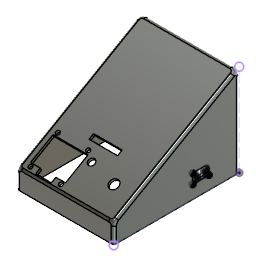
Morse Keyer Top Shell (Autodesk Fusion 360 design; units mm, degrees)
part number: 2026-05-24-21-26-59-922
Autodesk Fusion 360 part; units mm, degrees
sketch "Sketch1" plane through (0, 0, 0) normal (0, 0, 1) x (1, 0, 0)
  line L0 (37.5, 48.5) -> (-37.5, 48.5)
  line L1 (-37.5, 48.5) -> (-37.5, -48.5)
  line L2 (-37.5, -48.5) -> (37.5, -48.5)
  line L3 (37.5, -48.5) -> (37.5, 48.5)
  line L4 (37.5, 48.5) -> (-37.5, -48.5) construction
  line L5 (-37.5, 48.5) -> (37.5, -48.5) construction
  dimension "d1" = 75
  dimension "d2" = 97
  constraint horizontal L0
  constraint perpendicular L0 L1
  constraint parallel L0 L2
  constraint parallel L1 L3
  constraint coincident L4 origin
  constraint coincident L5 origin
  measures "d1" distance of L1.end L2.end
  measures "d2" distance of L0.end L1.end
extrude "Extrude1" add sketch "Sketch1" along normal blind 15
sketch "Sketch2" plane through (37.5, 0, 0) normal (1, 0, 0) x (0, 1, 0)
  line L0 (-48.5, 0) -> (48.5, 0)
  line L1 (48.5, 0) -> (48.5, 15)
  line L2 (48.5, 15) -> (-48.5, 15)
  line L3 (-48.5, 15) -> (-48.5, 0)
  line L4 (-48.5, 15) -> (48.5, 71.003)
  line L5 (-48.5, 15) -> (74.9401, 15) construction
  line L6 (48.5, 71.003) -> (48.5, 15)
  dimension "d5" = 30
  constraint horizontal L5
  constraint coincident L2.end L3.start
  constraint coincident L1.end L2.start
  constraint parallel L1 L6
  measures "d5" angle of L4 L5
extrude "Extrude2" add sketch "Sketch2" against normal up to surface (75 mm away) contours L2 L4 L6
sketch "Sketch3" plane through (0, -18.6202, 32.2511) normal (0, -0.5, 0.866025) x (1, 0, 0)
  line L0 (-37.5, 77.5037) -> (-37.5, -34.5022)
  line L1 (-37.5, -34.5022) -> (37.5, -34.5022)
  line L2 (37.5, -34.5022) -> (37.5, 77.5037)
  line L3 (37.5, 77.5037) -> (-37.5, 77.5037)
  line L4 (11, 3.5037) -> (-11, 3.5037)
  line L5 (-11, 3.5037) -> (-11, -0.4963)
  line L6 (-11, -0.4963) -> (11, -0.4963)
  line L7 (11, -0.4963) -> (11, 3.5037)
  line L8 (11, 3.5037) -> (-11, -0.4963) construction
  line L9 (-11, 3.5037) -> (11, -0.4963) construction
  line L10 (-32, -32.5022) -> (-5, -32.5022)
  line L11 (-5, -32.5022) -> (-5, -8.5022)
  line L12 (-5, -8.5022) -> (-32, -8.5022)
  line L13 (-32, -8.5022) -> (-32, -32.5022)
  circle A0 centre (-30.25, -6.2022) radius 1.5
  circle A1 centre (-6.75, -6.2022) radius 1.5
  circle A2 centre (21.25, -15.4993) radius 3.5
  line L14 (-32, -32.5022) -> (-24.5, -32.5022)
  line L15 (-24.5, -32.5022) -> (-24.5, -28.5022)
  line L16 (-24.5, -28.5022) -> (-32, -28.5022)
  line L17 (-32, -28.5022) -> (-32, -32.5022)
  line L18 (-5, -32.5022) -> (-12.5, -32.5022)
  line L19 (-12.5, -32.5022) -> (-12.5, -28.5022)
  line L20 (-12.5, -28.5022) -> (-5, -28.5022)
  line L21 (-5, -28.5022) -> (-5, -32.5022)
  circle A3 centre (-6.75, -30.5022) radius 1.5
  circle A4 centre (-30.25, -30.5022) radius 1.5
  line L22 (11, 3.5037) -> (37.5, 3.5037) construction
  line L23 (-11, 3.5037) -> (-37.5, 3.5037) construction
  line L24 (21.25, 3.5037) -> (21.25, -34.5022) construction
  circle A5 centre (0, -11.0022) radius 2.5
  line L25 (-5, -8.5022) -> (6, -8.5022) construction
  point P0 (0, 1.5037)
  dimension "d8" = 22
  dimension "d9" = 4
  dimension "d10" = 74
  dimension "d11" = 27
  dimension "d12" = 24
  dimension "d14" = 2
  dimension "d17" = 3
  dimension "d18" = 2.3
  dimension "d20" = 2.3
  dimension "d22" = 7
  dimension "d37" = 3
  dimension "d38" = 7.5
  dimension "d39" = 4
  dimension "d40" = 7.5
  dimension "d41" = 4
  dimension "d42" = 3
  dimension "d43" = 2
  dimension "d44" = 1.75
  dimension "d45" = 23.5
  dimension "d46" = 24.3
  dimension "d54" = 1.75
  dimension "d55" = 1.75
  dimension "d56" = 16.25
  dimension "d57" = 5
  dimension "d58" = 5
  constraint horizontal L4
  constraint perpendicular L4 L5
  constraint parallel L4 L6
  constraint parallel L5 L7
  constraint coincident L8 P0
  constraint coincident L9 P0
  constraint horizontal L10
  constraint vertical L11
  constraint horizontal L12
  constraint vertical L13
  constraint horizontal L14
  constraint vertical L15
  constraint horizontal L16
  constraint vertical L17
  constraint horizontal L18
  constraint vertical L19
  constraint horizontal L20
  constraint vertical L21
  constraint coincident L2 L22.end
  constraint perpendicular L2 L22
  constraint coincident L0 L23.end
  constraint perpendicular L0 L23
  constraint coincident L22 L24.start
  constraint coincident L1 L24.end
  constraint perpendicular L1 L24
  constraint midpoint A2.centre L24
  constraint perpendicular L11 L25
  constraint tangent A5 L25
  measures "d8" distance of L5.end L6.end
  measures "d9" distance of L4.end L5.end
  measures "d10" distance of L3 L4
  measures "d11" distance of L10.start L10.end
  measures "d12" distance of L10.start L12.end
  measures "d14" distance of L1 L10
  measures "d17" diameter of A0
  measures "d18" distance of L12 A0.centre
  measures "d20" distance of L12 A1.centre
  measures "d22" diameter of A2
  measures "d37" diameter of A1
  measures "d38" distance of L10.start L14.end
  measures "d39" distance of L10.start L16.end
  measures "d40" distance of L10.end L18.end
  measures "d41" distance of L10.end L20.end
  measures "d42" diameter of A3
  measures "d43" distance of L20 A3.centre
  measures "d44" distance of L11 A3.centre
  measures "d45" distance of A0.centre A1.centre
  measures "d46" distance of A0.centre A4.centre
  measures "d54" distance of L13 A0.centre
  measures "d55" distance of L13 A4.centre
  measures "d56" distance of L2 L24
  measures "d57" diameter of A5
  measures "d58" distance of L11 A5.centre
shell "Shell1" thickness 2 removed faces 1 at (-12.5, -16.1667, 0)
extrude "Extrude3" cut sketch "Sketch3" against normal blind 14 contours L4 L5 L6 L7 | L10 L11 L12 L13 L15 L16 L19 L20 | A0 | A1 | A2 | A3 | A4 | A5
sketch "Sketch4" plane through (37.5, 0, 0) normal (1, 0, 0) x (0, 1, 0)
  line L0 (-48.5, 0) -> (48.5, 0)
  line L1 (48.5, 0) -> (48.5, 71.003)
  line L2 (48.5, 71.003) -> (-48.5, 15)
  line L3 (-48.5, 15) -> (-48.5, 0)
sketch "Sketch5" plane through (37.5, 0, 0) normal (1, 0, 0) x (0, 1, 0)
  line L0 (15.5, 10.25) -> (22, 10.25)
  line L1 (25, 13.25) -> (25, 14.75)
  line L2 (22, 17.75) -> (15.5, 17.75)
  line L3 (12.5, 14.75) -> (12.5, 13.25)
  arc A0 (15.5, 17.75) -> (12.5, 14.75) centre (15.5, 14.75) ccw
  arc A1 (12.5, 13.25) -> (15.5, 10.25) centre (15.5, 13.25) ccw
  arc A2 (25, 14.75) -> (22, 17.75) centre (22, 14.75) ccw
  arc A3 (22, 10.25) -> (25, 13.25) centre (22, 13.25) ccw
  line L4 (18.75, 17.75) -> (18.75, 10.25) construction
  line L5 (12.5, 14) -> (25, 14) construction
  line L6 (-48.5, 0) -> (48.5, 0) construction
  line L7 (48.5, 0) -> (48.5, 71.003) construction
  point P0 (12.5, 10.25)
  point P1 (25, 10.25)
  point P2 (12.5, 17.75)
  dimension "d28" = 12.5
  dimension "d29" = 7.5
  dimension "d30" = 3
  dimension "d31" = 14
  dimension "d32" = 29.75
  constraint horizontal L0
  constraint vertical L1
  constraint horizontal L2
  constraint vertical L3
  constraint coincident P2 L2
  constraint coincident P2 L3
  constraint tangent L2 A0
  constraint tangent L3 A0
  constraint coincident P0 L0
  constraint coincident P0 L3
  constraint tangent L0 A1
  constraint tangent L3 A1
  constraint equal A0 A1
  constraint tangent L1 A2
  constraint tangent L2 A2
  constraint equal A0 A2
  constraint coincident P1 L0
  constraint coincident P1 L1
  constraint tangent L0 A3
  constraint tangent L1 A3
  constraint equal A0 A3
  constraint midpoint L2 L4.start
  constraint midpoint L0 L4.end
  constraint midpoint L3 L5.start
  constraint midpoint L1 L5.end
  measures "d28" distance of P0 P1
  measures "d29" distance of P0 P2
  measures "d30" radius of A0
  measures "d31" distance of L5 L6
  measures "d32" distance of L4 L7
extrude "Extrude4" cut sketch "Sketch5" against normal blind 4
fillet "Fillet1" radius 2 8 edges at (0, 48.5, 71.003) (-37.5, 0, 43.0015) (0, -48.5, 15) (-37.5, -48.5, 7.5) (-37.5, 48.5, 35.5015) (37.5, 0, 43.0015) (37.5, -48.5, 7.5) (37.5, 48.5, 35.5015)
